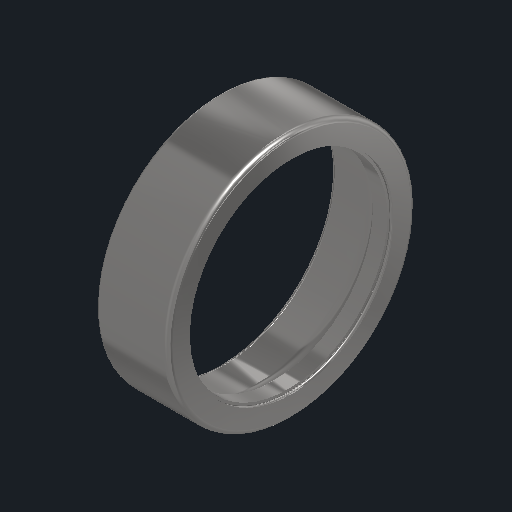
# Autodesk Inventor part: SKF_7205 BE-2RZP_PART2
Saved by Autodesk Inventor 2022 (Build 260153000, 153)
## iProperties
Part Number: SKF_7205 BE-2RZP_PART2
Material: Stainless Steel, 440C
Catalog Web Link: www.cadenas.de
Description: -Angular contact ball bearings, single row
Vendor: SKF
Document SubType Name: Modeling
Designer: partserver
Manufacturer: SKF
Mass: 130 g
Surface Area: 58.8054 cm^2
Volume: 7.83783 cm^3
Density: 7.75 g/cm^3
Appearance: Semi-Polished
Category: PARTsolutions
Company: SKF
PSOL_IDENT_0: {$CADENAS_DATA\23d-libs\skf\bearings_units_and_housings\ball_bearings\angular_contact_ball_bearings\
PSOL_IDENT_1: ba1_001_101.prj},212 {VTYP=3D},{NB=SKF_7205 BE-2RZP_PART2},{LINA=SKF_7205 BE-2RZP_PART2},{NN=BA1_001
PSOL_IDENT_2: _101_PART2},{NOPRJ=TRUE},{DATE=13.09.2021 11:18:32},{GEOMDATE=07.09.2021 05:50:45},{VERSION=},{LINEI
PSOL_IDENT_3: D=141990},{WBVAR=},{WBNUMERIC=}  {NB=SKF_7205 BE-2RZP_PART2},{LINA=SKF_7205 BE-2RZP_PART2},{KT=DUMMY
PSOL_IDENT_4: },{DESIGNATION=7205 BE-2RZP},{DD=25.000},{D=52.000},{B=15.0000},{DD1=35.850},{DD2=30.870},{D1=41.570
PSOL_IDENT_5: },{D2=42.700},{D3=MIN},{D4=46.270},{D5=46.8},{C1=MIN},{AA=24},{R12=1.000},{R34=0.600},{ALPHA=40},{PI
PSOL_IDENT_6: TCH=38.500},{DW=7.938},{DDAMIN=30.6},{DDAMAX=35.5},{DAMAX=46.4},{DBMAX=47.8},{RAMAX=1},{RBMAX=0.6},{
PSOL_IDENT_7: LOAD1=14.8},{LOAD2=9.3},{LOAD3=0.4},{SPEED1=16000},{SPEED2=12000},{Z=13},{II=1},{MASS=0.13},{BEARING=
PSOL_IDENT_8: 7205 BE-2RZP},{POPULAR=Yes},{VARIANT=design_ba1_001_101_1},{D2A=42.7},{DD2A=30.870},{R5R=0.6},{R34L=
PSOL_IDENT_9: 1},{IRH=1},{ORH=1},{D4H=1}
NB: SKF_7205 BE-2RZP_PART2
NT: Angular contact ball bearings, single row
NBSYN: SKF_$DESIGNATION._PART2
LINA: SKF_7205 BE-2RZP_PART2
CATALOG: SKF
DESIGNATION: 7205 BE-2RZP
DD: 25
D: 52
B: 15
LOAD1: 14.8
LOAD2: 9.3
LOAD3: 0.4
SPEED1: 16000
SPEED2: 12000
BEARING: 7205 BE-2RZP
SUPPLIER: SKF
ARTICLENO: SKF_7205 BE-2RZP_PART2
BOMINFO: SKF_7205 BE-2RZP_PART2
CREATOR: CADENAS GmbH
Title: SKF_7205 BE-2RZP_PART2
Author: Cadenas PARTsolutions
Comments: Angular contact ball bearings, single row
Autodesk Inventor part; units mm, degrees
ref_plane "YZ Plane" through (0, 0, 0) normal (1, 0, 0) x (0, 1, 0)
ref_plane "XZ Plane" through (0, 0, 0) normal (0, 1, 0) x (-1, 0, 0)
ref_plane "XY Plane" through (0, 0, 0) normal (0, 0, 1) x (1, 0, 0)
sketch "Sketch_4" plane through (0, 0, 0) normal (0, 0, 1) x (1, 0, 0)
  line L0 (15, 0) -> (0, 0)
  line L1 (0, 25) -> (0, 21.35)
  line L2 (0, 21.35) -> (0.1667, 21.35)
  arc A0 (0.8333, 21.35) -> (0.1667, 21.35) centre (0.5, 21.35) ccw
  line L3 (0.8333, 21.35) -> (0.8333, 20.885)
  line L4 (0.8333, 20.885) -> (3.8834, 20.885)
  arc A1 (7.5, 23.219) -> (3.8834, 20.885) centre (7.5, 19.25) ccw
  line L5 (7.5, 23.219) -> (14.1667, 23.219)
  line L6 (14.1667, 23.219) -> (14.1667, 23.675)
  arc A2 (14.8333, 23.675) -> (14.1667, 23.675) centre (14.5, 23.675) ccw
  line L7 (14.8333, 23.675) -> (15, 23.675)
  line L8 (15, 23.675) -> (15, 25.4)
  arc A3 (15, 25.4) -> (14.4, 26) centre (14.4, 25.4) ccw
  line L9 (14.4, 26) -> (1, 26)
  arc A4 (1, 26) -> (0, 25) centre (1, 25) ccw
  constraints: 20 end point, 10 point on circle, 5 centre point
revolve "Revolution1" add sketch "Sketch_4" angle 360 about axis through (15, 0, 0) along (1, 0, 0)
body "Solid1"
